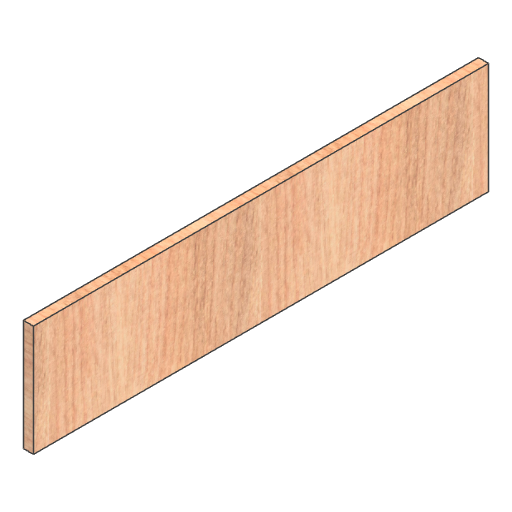
# Autodesk Inventor part: CUT PART O-01
Saved by Autodesk Inventor 2023.2 (Build 272271000, 271)
## iProperties
Created: 2022-11-08
Part Number: CUT PART O-01
Material: Wood (Birch)
Document SubType Name: Modeling
Designer: GUT
Density: 0.55 g/cm^3
Appearance: Birch - Natural Polished
Mass: 478.401 g
Surface Area: 1612.42 cm^2
Volume: 869.82 cm^3
d0: 133,000 mm
Author: GUT
Autodesk Inventor part; units mm, degrees
ref_plane "YZ Plane" through (0, 0, 0) normal (1, 0, 0) x (0, 1, 0)
ref_plane "XZ Plane" through (0, 0, 0) normal (0, 1, 0) x (-1, 0, 0)
ref_plane "XY Plane" through (0, 0, 0) normal (0, 0, 1) x (1, 0, 0)
sketch "Sketch1" plane through (0, 0, 0) normal (1, 0, 0) x (0, 1, 0)
  line L0 (15.288, -124.9899) -> (148.288, -124.9899)
  line L1 (148.288, -124.9899) -> (148.288, -669.9899)
  line L2 (148.288, -669.9899) -> (15.288, -669.9899)
  line L3 (15.288, -669.9899) -> (15.288, -124.9899)
  point P0 (0, 0)
  dimension "d0" = 133
  dimension "b" = 545
  constraints: 8 end point, 2 parallel, 1 horizontal, 1 perpendicular
  measures "d0" distance of L1.end L2.end
  measures "b" distance of L0.end L1.end
extrude "Extrusion1" add sketch "Sketch1" along normal blind 12
body "Solid1"
